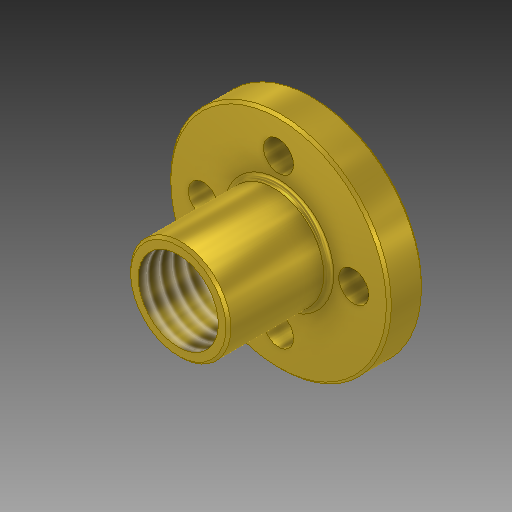
# Autodesk Inventor part: Tuerca_Tornillo de potencia
Saved by Autodesk Inventor 2019 (Build 230136000, 136)
## iProperties
Created: 2018-08-31
Part Number: Tuerca_Tornillo de potencia
Material: Generic
Document SubType Name: Modeling
Designer: Jurgen
Density: 1 g/cm^3
Appearance: Metal 2400F Hot
Mass: 1.39134 g
Surface Area: 17.1187 cm^2
Volume: 1.39134 cm^3
Author: Jurgen
Autodesk Inventor part; units mm, degrees
ref_plane "YZ Plane" through (0, 0, 0) normal (1, 0, 0) x (0, 1, 0)
ref_plane "XZ Plane" through (0, 0, 0) normal (0, 1, 0) x (-1, 0, 0)
ref_plane "XY Plane" through (0, 0, 0) normal (0, 0, 1) x (1, 0, 0)
sketch "Sketch1" plane through (0, 0, 0) normal (0, 0, 1) x (1, 0, 0)
  circle A0 centre (0, 0) radius 11
  dimension "d0" = 22
  constraints: 1 centre point, 1 coincident
  measures "d0" diameter of A0
extrude "Extrusion1" add sketch "Sketch1" along normal blind 3.5
sketch "Sketch2" plane through (0, 0, 3.5) normal (0, 0, 1) x (1, 0, 0)
  circle A0 centre (0, 0) radius 5
  circle A1 centre (0, 0) radius 4
  dimension "d3" = 10
  dimension "d4" = 8
  constraints: 2 centre point, 2 coincident
  measures "d3" diameter of A0
  measures "d4" diameter of A1
extrude "Extrusion2" add sketch "Sketch2" along normal blind 10
sketch "Sketch3" plane through (0, 0, 3.5) normal (0, 0, 1) x (1, 0, 0)
  circle A0 centre (0, 0) radius 4
  dimension "d7" = 8
  constraints: 1 centre point, 1 coincident
  measures "d7" diameter of A0
extrude "Extrusion3" cut sketch "Sketch3" against normal blind 10
sketch "Sketch4" plane through (0, 0, 0) normal (0, 0, -1) x (-1, 0, 0)
  circle A0 centre (0, 0) radius 4 projected
  circle A1 centre (0, 0) radius 5
  dimension "d10" = 10
  constraints: 1 centre point, 1 coincident
  measures "d10" diameter of A1
extrude "Extrusion4" add sketch "Sketch4" along normal blind 2
fillet "Fillet1" radius 0.5 1 edges at (-5, 0, 3.5)
chamfer "Chamfer1" distance 0.25 angle 45 1 edges at (-5, 0, 13.5)
chamfer "Chamfer2" distance 0.25 angle 45 2 edges at (-11, 0, 3.5) (-11, 0, 0)
sketch "Sketch5" plane through (0, 0, 3.5) normal (0, 0, 1) x (1, 0, 0)
  circle A0 centre (0, 0) radius 11 construction
  circle A1 centre (0, 0) radius 7.5 construction
  circle A2 centre (0, 7.5) radius 1.5 construction
  circle A3 centre (0, 7.5) radius 1.5
  circle A4 centre (-7.5, 0) radius 1.5 construction
  circle A5 centre (-7.5, 0) radius 1.5
  circle A6 centre (0, -7.5) radius 1.5 construction
  circle A7 centre (0, -7.5) radius 1.5
  circle A8 centre (7.5, 0) radius 1.5 construction
  circle A9 centre (7.5, 0) radius 1.5
  dimension "d21" = 15
  dimension "d20" = 22
  dimension "d22" = 3
  dimension "d25" = 360
  constraints: 9 centre point, 6 coincident, 1 concentric, 1 vertical alignment, 19 other
  measures "d20" diameter of A0
  measures "d22" diameter of A2
extrude "Extrusion5" cut sketch "Sketch5" against normal through all
thread "Thread1" size "M8x1.25" class "6H" standard "ANSI Metric M Profile" full length
body "Solid1"
